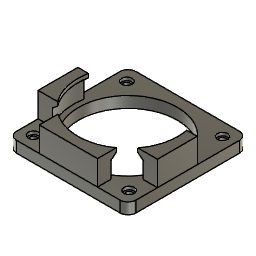
digiObscura Camera_LensMount v5 (Autodesk Fusion 360 design; units mm, degrees)
Autodesk Fusion 360 part; units mm, degrees
sketch "Sketch1" plane through (0, 0, 81.6) normal (0, 0, 1) x (1, 0, 0)
  ellipse E0 centre (50, -38.1356) end of major axis (50, -40.3423) minor radius 2 (50, -40.3423) -> (52, -38.1356) ccw
  line L0 (52, -38.1356) -> (52, 38.1356)
  ellipse E1 centre (50, 38.1356) end of major axis (50, 40.3423) minor radius 2 (52, 38.1356) -> (50, 40.3423) ccw
  line L1 (50, 40.3423) -> (-50, 40.3423)
  ellipse E2 centre (-50, 38.1356) end of major axis (-50, 40.3423) minor radius 2 (-50, 40.3423) -> (-52, 38.1356) ccw
  line L2 (-52, 38.1356) -> (-52, -38.1356)
  ellipse E3 centre (-50, -38.1356) end of major axis (-50, -40.3423) minor radius 2 (-52, -38.1356) -> (-50, -40.3423) ccw
  line L3 (-50, -40.3423) -> (50, -40.3423)
  circle A0 centre (30.0531, 29.3396) radius 2.1
  circle A1 centre (0, 0) radius 31
  circle A2 centre (30.0531, -29.3396) radius 2.1
  circle A3 centre (-30.0531, 29.3396) radius 2.1
  circle A4 centre (-30.0531, -29.3396) radius 2.1
  line L4 (32.5, -37.5) -> (-32.5, -37.5)
  line L5 (-37.5, -32.5) -> (-37.5, 32.5)
  line L6 (-32.5, 37.5) -> (32.5, 37.5)
  line L7 (37.5, 32.5) -> (37.5, -32.5)
  line L8 (37.5, -37.5) -> (-37.5, 37.5) construction
  line L9 (-37.5, -37.5) -> (37.5, 37.5) construction
  circle A5 centre (-30.0531, -29.3396) radius 1.75
  line L10 (0, 0) -> (-16, 0) construction
  line L11 (0, 0) -> (0, 14) construction
  circle A6 centre (-30.0531, 29.3396) radius 1.75
  circle A7 centre (30.0531, 29.3396) radius 1.75
  circle A8 centre (30.0531, -29.3396) radius 1.75
  arc A9 (-37.5, -32.5) -> (-32.5, -37.5) centre (-32.5, -32.5) ccw
  arc A10 (-32.5, 37.5) -> (-37.5, 32.5) centre (-32.5, 32.5) ccw
  arc A11 (37.5, 32.5) -> (32.5, 37.5) centre (32.5, 32.5) ccw
  arc A12 (32.5, -37.5) -> (37.5, -32.5) centre (32.5, -32.5) ccw
  dimension "d135" = 75
  dimension "d136" = 75
  dimension "d137" = 3.5
  dimension "d138" = 5
  dimension "d139" = 5
  dimension "d140" = 5
  dimension "d141" = 5
  dimension "d1" = 42
  constraint perpendicular L4 L5
  constraint parallel L4 L6
  constraint parallel L5 L7
  constraint horizontal L4
  constraint coincident L8 A1.centre
  constraint coincident L9 A1.centre
  constraint coincident A1.centre L10.start
  constraint concentric A4 A5
  constraint perpendicular L7 L10
  constraint perpendicular L10 L11
  constraint symmetric A5 L10 A6
  constraint symmetric A5 L11 A8
  constraint symmetric L11 A6 A7
  constraint coincident L9.start L4
  constraint coincident L9.start L5
  constraint tangent L4 A9
  constraint tangent L5 A9
  constraint coincident L8.end L5
  constraint coincident L8.end L6
  constraint tangent L5 A10
  constraint tangent L6 A10
  constraint coincident L9.end L6
  constraint coincident L9.end L7
  constraint tangent L6 A11
  constraint tangent L7 A11
  constraint coincident L8.start L7
  constraint coincident L8.start L4
  constraint tangent L7 A12
  constraint tangent L4 A12
  constraint coincident A3.centre A6.centre
  constraint coincident A0.centre A7.centre
  constraint coincident A2.centre A8.centre
  measures "d135" distance of L8.start L9.start
  measures "d136" distance of L8.start L9.end
  measures "d137" diameter of A5
  measures "d138" radius of A9
  measures "d139" radius of A10
  measures "d140" radius of A11
  measures "d141" radius of A12
  measures "d1" distance of A1.centre A4.centre
extrude "Extrude1" add sketch "Sketch1" along normal blind 7 contours L4 L5 L6 L7 A9 A10 A11 A12 makes body 1
sketch "Sketch2" plane through (0, 0, 88.6) normal (0, 0, 1) x (1, 0, 0)
  circle A0 centre (30.0531, -29.3396) radius 2.1
  circle A1 centre (-30.0531, -29.3396) radius 2.1
  circle A2 centre (0, 0) radius 31
  circle A3 centre (30.0531, 29.3396) radius 2.1
  circle A4 centre (-30.0531, 29.3396) radius 2.1
  arc A5 (-37.5, -32.5) -> (-32.5, -37.5) centre (-32.5, -32.5) ccw
  line L0 (-32.5, -37.5) -> (32.5, -37.5)
  arc A6 (32.5, -37.5) -> (37.5, -32.5) centre (32.5, -32.5) ccw
  line L1 (37.5, -32.5) -> (37.5, 32.5)
  arc A7 (37.5, 32.5) -> (32.5, 37.5) centre (32.5, 32.5) ccw
  line L2 (32.5, 37.5) -> (-32.5, 37.5)
  arc A8 (-32.5, 37.5) -> (-37.5, 32.5) centre (-32.5, 32.5) ccw
  line L3 (-37.5, 32.5) -> (-37.5, -32.5)
  circle A9 centre (-30.0531, -29.3396) radius 3.25
  line L4 (0, 0) -> (-10, 0) construction
  line L5 (0, 0) -> (0, 11) construction
  circle A10 centre (-30.0531, 29.3396) radius 3.25
  circle A11 centre (30.0531, 29.3396) radius 3.25
  circle A12 centre (30.0531, -29.3396) radius 3.25
  dimension "d144" = 6.5
  constraint concentric A1 A9
  constraint coincident A2.centre L4.start
  constraint perpendicular L1 L4
  constraint perpendicular L4 L5
  constraint symmetric A9 L4 A10
  constraint symmetric A9 L5 A12
  constraint symmetric L5 A10 A11
  measures "d144" diameter of A9
extrude "Extrude2" cut sketch "Sketch2" against normal blind 2 contours A9 | A10 | A11 | A12 bodies 1
sketch "Sketch3" plane through (0, 0, 88.6) normal (0, 0, 1) x (1, 0, 0)
  arc A0 (-37.5, -32.5) -> (-32.5, -37.5) centre (-32.5, -32.5) ccw
  line L0 (-32.5, -37.5) -> (32.5, -37.5)
  arc A1 (32.5, -37.5) -> (37.5, -32.5) centre (32.5, -32.5) ccw
  line L1 (37.5, -32.5) -> (37.5, 32.5)
  arc A2 (37.5, 32.5) -> (32.5, 37.5) centre (32.5, 32.5) ccw
  line L2 (32.5, 37.5) -> (-32.5, 37.5)
  arc A3 (-32.5, 37.5) -> (-37.5, 32.5) centre (-32.5, 32.5) ccw
  line L3 (-37.5, 32.5) -> (-37.5, -32.5)
  circle A4 centre (-30.0531, 29.3396) radius 3.25
  circle A5 centre (30.0531, 29.3396) radius 3.25
  circle A6 centre (30.0531, -29.3396) radius 3.25
  circle A7 centre (-30.0531, -29.3396) radius 3.25
  circle A8 centre (0, 0) radius 34.25
  line L4 (33.7204, 6) -> (37.5, 6)
  line L5 (37.5, 6) -> (37.5, -19)
  line L6 (37.5, -19) -> (28.4967, -19)
  line L7 (0, 0) -> (0, -14) construction
  line L8 (18.3174, -28.9402) -> (18.3174, -37.5)
  line L9 (0, -37.5) -> (18.3174, -37.5)
  line L10 (0, -37.5) -> (-18.3174, -37.5)
  line L11 (-18.3174, -28.9402) -> (-18.3174, -37.5)
  line L12 (-33.7204, 6) -> (-37.5, 6)
  line L13 (-37.5, 6) -> (-37.5, -19)
  line L14 (-37.5, -19) -> (-28.4967, -19)
  circle A9 centre (0, 0) radius 31
  dimension "d153" = 68.5
  dimension "d2" = 6
  constraint concentric A8 A9
  constraint coincident A8 L4.start
  constraint coincident L1 L4.end
  constraint perpendicular L1 L4
  constraint coincident L1 L5.end
  constraint coincident A8 L6.end
  constraint perpendicular L5 L6
  constraint coincident A8.centre L7.start
  constraint perpendicular L4 L7
  constraint coincident A8 L8.start
  constraint coincident L0 L8.end
  constraint perpendicular L0 L8
  constraint midpoint L0 L9.start
  constraint symmetric L7 L8.start L11.start
  constraint symmetric L7 L8.end L10.end
  constraint symmetric L7 L9.start L10.start
  constraint symmetric L4.start L7 L12.start
  constraint symmetric L4.end L7 L12.end
  constraint symmetric L5.end L7 L13.end
  constraint symmetric L6.end L7 L14.end
  measures "d153" diameter of A8
  measures "d2" distance of A8.centre L4
extrude "Extrude3" add sketch "Sketch3" along normal blind 10.5 separate body contours L3 A8 L12 L13 L14 | L0 A8 L8 L9 L10 L11 | L1 A8 L4 L5 L6 makes body 2 at (-32.8111, -9.823, 95.6) makes body 3 at (-11.0715, -32.4112, 95.6) makes body 4 at (33.9446, 4.5635, 95.6)
sketch "Sketch4" plane through (0, 0, 99.1) normal (0, 0, 1) x (1, 0, 0)
  line L0 (-33.7204, 6) -> (-37.5, 6)
  line L1 (-37.5, 6) -> (-37.5, -19)
  line L2 (-37.5, -19) -> (-28.4967, -19)
  arc A0 (-33.7204, 6) -> (-28.4967, -19) centre (0, 0) ccw
  circle A1 centre (0, 0) radius 31.5
  line L3 (-37.5, 6) -> (-30.9233, 6)
  line L4 (-37.5, -19) -> (-25.1247, -19)
  line L5 (-18.3174, -25.6266) -> (-18.3174, -37.5)
  line L6 (18.3174, -25.6266) -> (18.3174, -37.5)
  line L7 (30.9233, 6) -> (37.5, 6)
  line L8 (25.1247, -19) -> (37.5, -19)
  line L9 (-18.3174, -37.5) -> (18.3174, -37.5)
  line L10 (37.5, -19) -> (37.5, 6)
  point P0 (-18.3174, -37.5)
  point P1 (18.3174, -37.5)
  point P2 (37.5, -19)
  point P3 (37.5, 6)
  dimension "d150" = 63
  constraint concentric A0 A1
  constraint coincident L0.end L1.start
  constraint coincident A1 L3.end
  constraint perpendicular L1 L3
  constraint coincident L1.end L2.start
  constraint coincident A1 L4.end
  constraint perpendicular L1 L4
  constraint coincident A1 L5.start
  constraint vertical L5
  constraint coincident A1 L6.start
  constraint vertical L6
  constraint coincident L5 P0
  constraint coincident L6 P1
  constraint coincident A1 L7.start
  constraint horizontal L7
  constraint coincident A1 L8.start
  constraint horizontal L8
  constraint coincident L8 P2
  constraint coincident L7 P3
  constraint coincident P0 L5.end
  constraint coincident P1 L6.end
  constraint coincident P2 L8.end
  constraint coincident P3 L7.end
  measures "d150" diameter of A1
extrude "Extrude4" add sketch "Sketch4" along normal blind 5 contours L0 L1 L2 A0 L3 L4 | A0 A1 L3 L4 | A1 L7 L8 L10 | A1 L5 L6 L9 bodies 2 3 4
chamfer "Chamfer1" distance 2.6 angle 45 1 edges at (-30.6854, -7.1173, 99.1) on bodies 2
chamfer "Chamfer2" distance 2.6 angle 45 1 edges at (0, -31.5, 99.1) on bodies 3
chamfer "Chamfer3" distance 2.6 angle 45 1 edges at (30.6854, -7.1173, 99.1) on bodies 4
equation "d148 = 11.7 mm - 1.2 mm"
